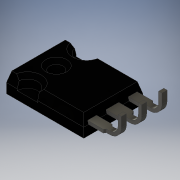
# Autodesk Inventor part: TO-247-Underheat
Saved by Autodesk Inventor 2016 (Build 200138000, 138)
## iProperties
Created: 2016-09-10
Part Number: TO-247-Underheat
Material: Generic
Document SubType Name: Modeling
Designer: jfixelle
Density: 1 g/cm^3
Appearance: Black
Author: jfixelle
Autodesk Inventor part; units mm, degrees
ref_plane "YZ Plane" through (0, 0, 0) normal (1, 0, 0) x (0, 1, 0)
ref_plane "XZ Plane" through (0, 0, 0) normal (0, 1, 0) x (-1, 0, 0)
sketch "Sketch1" plane through (0, 0, 0) normal (0, 1, 0) x (-1, 0, 0)
  line L0 (10.41, 7.935) -> (-10.41, 7.935)
  line L1 (-10.41, 7.935) -> (-10.41, -7.935)
  line L2 (-10.41, -7.935) -> (10.41, -7.935)
  line L3 (10.41, -7.935) -> (10.41, 7.935)
  point P0 (0, 0)
  dimension "d0" = 15.87
  dimension "d1" = 7.935
  dimension "d2" = 20.82
  dimension "d3" = 10.41
  constraints: 8 end point, 2 parallel, 1 horizontal, 1 perpendicular
  measures "d0" distance of L2.end L0.start
  measures "d1" distance from line of point (0, 0) L2
  measures "d2" distance of L1.end L2.end
  measures "d3" distance from line of point (0, 0) L3
extrude "Extrusion1" add sketch "Sketch1" along normal blind 5.31
chamfer "Chamfer1" distance 2.72 angle 15 1 edges at (0, 5.31, 7.935) measured on face at (-3.47, 1.77, 7.935)
chamfer "Chamfer2" distance 2.72 angle 15 1 edges at (10.41, 5.31, -0.3644) measured on face at (10.41, 3.54, -2.8879)
chamfer "Chamfer3" distance 2.72 angle 15 1 edges at (-0.3644, 5.31, -7.935) measured on face at (3.2271, 1.77, -7.935)
chamfer "Chamfer4" distance 2.72 angle 15 1 edges at (-10.41, 5.31, 0) measured on face at (-10.41, 3.4967, -2.4021)
sketch "Sketch3" plane through (0, 0, 0) normal (0, -1, 0) x (1, 0, 0)
  line L0 (-9.11, 6.86) -> (3.97, 6.86)
  line L1 (3.97, 6.86) -> (3.97, -6.86)
  line L2 (3.97, -6.86) -> (-9.11, -6.86)
  line L3 (-9.11, -6.86) -> (-9.11, 6.86)
  line L4 (-10.41, -7.935) -> (-10.41, 7.935) projected
  point P0 (0, 0)
  dimension "d20" = 13.08
  dimension "d21" = 13.72
  dimension "d22" = 6.86
  dimension "d23" = 1.3
  constraints: 8 end point, 2 parallel, 1 horizontal, 1 perpendicular
  measures "d20" distance of L1.end L2.end
  measures "d21" distance of L0.end L1.end
  measures "d22" distance from line of point (0, 0) L0
  measures "d23" distance between parallel lines of L4 L3
extrude "Extrusion2" add sketch "Sketch3" along normal blind 0.01
sketch "Sketch2" plane through (0, 5.31, 0) normal (0, 1, 0) x (1, 0, 0)
  circle A0 centre (-4.9, 0) radius 1.83
  line L0 (-10.41, 7.935) -> (-10.41, -7.935) projected
  point P0 (0, 0)
  dimension "d18" = 5.51
  dimension "d19" = 3.66
  constraints: 1 centre point
  measures "d18" distance from line of A0.centre L0
  measures "d19" diameter of A0
extrude "Extrusion3" cut sketch "Sketch2" against normal through all
sketch "Sketch4" plane through (0, 5.31, 0) normal (0, 1, 0) x (1, 0, 0)
  line L0 (-10.41, 7.935) -> (-10.41, -7.935) projected
  line L1 (-10.41, -7.935) -> (10.41, -7.935) projected
  line L2 (-9.3708, -7.935) -> (-0.6355, -7.935)
  circle A0 centre (-4.72, -7.935) radius 2.745
  point P0 (0, 0)
  dimension "d30" = 5.49
  dimension "d31" = 5.69
  constraints: 3 point on line, 2 end point, 1 centre point
  measures "d30" diameter of A0
  measures "d31" distance from line of L0 A0.centre
extrude "Extrusion4" cut sketch "Sketch4" against normal blind 3.14
mirror "Mirror1" about plane through (0, 0, 0) normal (0, 0, 1) of "Extrusion4"
chamfer "Chamfer5" distance 1 angle 45 3 edges at (-4.72, 5.31, 5.19) (-6.73, 5.31, 0) (-4.72, 5.31, -5.19)
ref_plane "Work Plane1" through (0, 2.59, 0) normal (0, -1, 0) x (1, 0, 0)
sketch "Sketch5" plane through (0, 2.59, 0) normal (0, -1, 0) x (1, 0, 0)
  line L0 (9.0645, 1.715) -> (14.7, 1.715)
  line L1 (14.7, 1.715) -> (14.7, -1.715)
  line L2 (14.7, -1.715) -> (9.0645, -1.715)
  line L3 (9.0645, -1.715) -> (9.0645, 1.715)
  line L4 (10.41, 7.935) -> (10.41, -7.935) projected
  line L5 (10.41, 0) -> (13.4225, 0)
  line L6 (10.1151, 6.655) -> (14.7, 6.655)
  line L7 (14.7, 6.655) -> (14.7, 4.265)
  line L8 (14.7, 4.265) -> (10.1151, 4.265)
  line L9 (10.1151, 4.265) -> (10.1151, 6.655)
  line L10 (14.7, 5.46) -> (14.8506, 5.46)
  line L11 (14.7, 6.16) -> (14.4142, 6.655)
  line L12 (14.7, 4.76) -> (14.4142, 4.265)
  line L13 (14.7, 0.7) -> (14.114, 1.715)
  line L14 (14.7, -0.7) -> (14.114, -1.715)
  line L15 (10.1151, -6.655) -> (14.7, -6.655)
  line L16 (14.7, -6.655) -> (14.7, -4.265)
  line L17 (14.7, -4.265) -> (10.1151, -4.265)
  line L18 (10.1151, -4.265) -> (10.1151, -6.655)
  line L19 (14.7, -6.16) -> (14.4142, -6.655)
  line L20 (14.7, -4.76) -> (14.4142, -4.265)
  point P0 (0, 0)
  dimension "d38" = 3.43
  dimension "d39" = 1.715
  dimension "d40" = 4.29
  dimension "d41" = 0
  dimension "d42" = 2.39
  dimension "d43" = 5.46
  dimension "d44" = 1.4
  dimension "d45" = 0.7
  dimension "d46" = 1.4
  dimension "d47" = 0.7
  dimension "d48" = 30
  dimension "d49" = 30
  dimension "d50" = 30
  dimension "d51" = 30
  constraints: 40 end point, 12 point on line, 8 symmetric about line, 4 horizontal, 4 parallel, 2 midpoint, 2 perpendicular
  measures "d38" distance of L0.end L1.end
  measures "d39" distance between parallel lines of L5 L2
  measures "d40" distance between parallel lines of L4 L1
  measures "d41" distance between parallel lines of L1 L7
  measures "d42" distance of L6.end L7.end
  measures "d43" distance between parallel lines of L5 L10
  measures "d44" distance of L12.start L11.start
  measures "d45" distance from line of L12.start L10
  measures "d46" distance of L13.start L14.start
  measures "d47" distance from line of L5 L14.start
  measures "d48" angle of L7 L12
  measures "d49" angle of L7 L11
  measures "d50" angle of L1 L13
  measures "d51" angle of L1 L14
extrude "Extrusion5" add sketch "Sketch5" against normal blind 0.86 contours L17 L20 L16 L19 L15 L4 | L4 L15 L18 L17 | L8 L9 L6 L4 | L4 L6 L11 L7 L12 L8 | L13 L1 L14 L2 L4 L0 | L4 L2 L3 L0
sketch "Sketch6" plane through (14.7, 2.59, 0.7) normal (1, 0, 0) x (0, 0, -1)
  line L0 (-5.46, 0) -> (-5.46, 0.86) projected
  line L1 (-4.06, 0) -> (-4.06, 0.86) projected
  line L2 (-5.46, 0) -> (-4.06, 0)
  line L3 (-4.06, 0) -> (-4.06, 0.86)
  line L4 (-4.06, 0.86) -> (-5.46, 0.86)
  line L5 (-5.46, 0.86) -> (-5.46, 0)
  line L6 (0, 0) -> (0, 0.86) projected
  line L7 (1.4, 0) -> (1.4, 0.86) projected
  line L8 (0, 0) -> (1.4, 0)
  line L9 (1.4, 0) -> (1.4, 0.86)
  line L10 (1.4, 0.86) -> (0, 0.86)
  line L11 (0, 0.86) -> (0, 0)
  line L12 (5.46, 0) -> (5.46, 0.86) projected
  line L13 (4.965, 0.86) -> (7.355, 0.86) projected
  line L14 (5.46, 0) -> (6.86, 0)
  line L15 (6.86, 0) -> (6.86, 0.86)
  line L16 (6.86, 0.86) -> (5.46, 0.86)
  line L17 (5.46, 0.86) -> (5.46, 0)
  point P0 (0.7, -2.59)
  dimension "d54" = 1.4
  constraints: 24 end point, 6 parallel, 3 horizontal, 3 perpendicular, 1 point on line
  measures "d54" distance of L15.end L16.end
sketch "Sketch7" plane through (0, 0, 0) normal (0, 0, 1) x (1, 0, 0)
  line L0 (14.7, 2.59) -> (14.7, 3.45) projected
  line L1 (14.7, 3.02) -> (15.6, 3.02)
  line L2 (18.3, 5.72) -> (18.3, 8.36)
  line L3 (10.41, 0) -> (-10.41, 0) projected
  arc A0 (15.6, 3.02) -> (18.3, 5.72) centre (15.6, 5.72) ccw
  point P0 (0, 0)
  point P1 (18.3, 3.02)
  dimension "d55" = 8.36
  dimension "d56" = 3.6
  dimension "d57" = 2.7
  constraints: 4 end point, 2 point on circle, 2 point on line, 2 tangent, 1 centre point, 1 horizontal, 1 midpoint, 1 perpendicular
  measures "d55" distance from line of L3 L2.end
  measures "d56" distance of L1.start point (18.3, 3.02)
  measures "d57" radius of A0
sweep "Sweep1" add profiles "Sketch6" path "Sketch7" path curves L1 A0 L2
body "Solid1"
